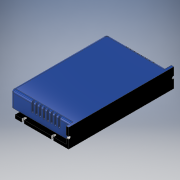
# Autodesk Inventor part: CopleyAccelus
Saved by Autodesk Inventor 2019 (Build 230136000, 136)
## iProperties
Created: 2019-05-13
Part Number: CopleyAccelus
Material: ABS Plastic
Document SubType Name: Modeling
Designer: Jorian Bruslind
Density: 1.06 g/cm^3
Appearance: Smooth - White
Author: Jorian Bruslind
Autodesk Inventor part; units mm, degrees
ref_plane "YZ Plane" through (0, 0, 0) normal (1, 0, 0) x (0, 1, 0)
ref_plane "XZ Plane" through (0, 0, 0) normal (0, 1, 0) x (-1, 0, 0)
sketch "Sketch1" plane through (0, 0, 0) normal (0, 1, 0) x (-1, 0, 0)
  line L0 (0, 0) -> (95, 0)
  line L1 (95, 0) -> (95, -152)
  line L2 (95, -152) -> (0, -152)
  line L3 (0, -152) -> (0, 0)
  dimension "d0" = 95
  dimension "d1" = 152
  constraints: 8 end point, 2 parallel, 1 horizontal, 1 perpendicular
  measures "d0" distance of L1.end L2.end
  measures "d1" distance of L0.end L1.end
extrude "Extrusion1" add sketch "Sketch1" along normal blind 25
sketch "Sketch2" plane through (0, 0, 0) normal (1, 0, 0) x (0, 0, -1)
  line L0 (0, 0) -> (0, -5)
  line L1 (0, -5) -> (-7.5, -5)
  line L2 (-7.5, -5) -> (159.5, -5)
  line L3 (159.5, -5) -> (159.5, 25)
  line L4 (159.5, 25) -> (-7.5, 25)
  line L5 (-7.5, 25) -> (-7.5, -5)
  point P0 (0, 25)
  dimension "d6" = 5
  dimension "d7" = 7.5
  dimension "d8" = 167
  dimension "d9" = 30
  constraints: 12 end point, 2 horizontal, 2 parallel, 1 perpendicular, 1 vertical
  measures "d6" distance of L0.start L0.end
  measures "d7" distance of L0.end L1.end
  measures "d8" distance of L4.end L3.end
  measures "d9" distance of L3.end L2.end
extrude "Extrusion2" add sketch "Sketch2" along normal blind 4
sketch "Sketch3" plane through (0, 0, 0) normal (-1, 0, 0) x (0, 0, 1)
  line L0 (7.5, 25) -> (7.5, -5) projected
  line L1 (-159.5, -5) -> (-159.5, 25) projected
  line L2 (7.5, -5) -> (-159.5, -5)
  line L3 (-159.5, -5) -> (-159.5, 0)
  line L4 (-159.5, 0) -> (7.5, 0)
  line L5 (7.5, 0) -> (7.5, -5)
  point P0 (0, 0)
  dimension "d12" = 5
  constraints: 8 end point, 2 parallel, 1 horizontal, 1 perpendicular, 1 point on line
  measures "d12" distance between parallel lines of L4 L2
extrude "Extrusion3" add sketch "Sketch3" along normal blind 81
sketch "Sketch4" plane through (4, -5, -159.5) normal (0, -1, 0) x (1, 0, 0)
  line L0 (-85, 0) -> (0, 0) projected
  line L1 (-85, 0) -> (-74.4, 0)
  line L2 (-74.4, 0) -> (-74.4, 3.5)
  arc A0 (-70.4, 3.5) -> (-74.4, 3.5) centre (-72.4, 3.5) ccw
  line L3 (-70.4, 3.5) -> (-70.4, 0)
  line L4 (-74.4, 0) -> (-70.4, 0)
  line L5 (-85, 0) -> (-85, 4)
  line L6 (-85, 0) -> (-85, 167) projected
  line L7 (-27.7, 0) -> (-27.7, 3.5)
  arc A1 (-23.7, 3.5) -> (-27.7, 3.5) centre (-25.7, 3.5) ccw
  line L8 (-23.7, 3.5) -> (-23.7, 0)
  line L9 (-27.7, 0) -> (-23.7, 0)
  line L10 (0, 0) -> (0, 167) projected
  line L11 (0, 0) -> (0, 83.5)
  line L12 (0, 83.5) -> (-10, 83.5)
  line L13 (-74.4, 167) -> (-74.4, 163.5)
  arc A2 (-74.4, 163.5) -> (-70.4, 163.5) centre (-72.4, 163.5) ccw
  line L14 (-70.4, 163.5) -> (-70.4, 167)
  line L15 (-74.4, 167) -> (-70.4, 167)
  line L16 (-27.7, 167) -> (-27.7, 163.5)
  arc A3 (-27.7, 163.5) -> (-23.7, 163.5) centre (-25.7, 163.5) ccw
  line L17 (-23.7, 163.5) -> (-23.7, 167)
  line L18 (-27.7, 167) -> (-23.7, 167)
  point P0 (-4, 159.5)
  dimension "d15" = 10.6
  dimension "d16" = 3.5
  dimension "d17" = 2
  dimension "d18" = 2
  dimension "d19" = 3.5
  dimension "d20" = 4
  dimension "d23" = 46.7
  dimension "d28" = 10
  constraints: 32 end point, 10 symmetric about line, 8 point on circle, 4 centre point, 3 point on line, 2 horizontal, 2 perpendicular, 1 midpoint, 1 vertical, 11 other
  measures "d15" distance of L0.start L1.end
  measures "d16" distance of L1.end L2.end
  measures "d17" radius of A0
  measures "d18" distance from line of L2 A0.centre
  measures "d19" distance of L3.start L3.end
  measures "d20" distance of L0.start L5.end
  measures "d23" distance of L1.end L7.start
  measures "d28" distance of L11.end L12.end
extrude "Extrusion4" cut sketch "Sketch4" against normal blind 5
fillet "Fillet1" radius 4 5 edges at (-47.5, 25, 0) (-47.5, 25, -152) (-95, 25, -76) (-95, 12.5, 0) (-95, 12.5, -152)
sketch "Sketch6" plane through (0, 25, 0) normal (0, 1, 0) x (1, 0, 0)
  line L0 (0, 0) -> (-18.5, 0)
  line L1 (-91, 0) -> (0, 0) projected
  line L2 (-18.5, 0) -> (-18.5, 1.5)
  arc A0 (-17, 1.5) -> (-20, 1.5) centre (-18.5, 1.5) ccw
  line L3 (-20, 1.5) -> (-20, 0)
  line L4 (-17, 1.5) -> (-17, 0)
  line L5 (-20, 0) -> (-17, 0)
  dimension "d41" = 18.5
  dimension "d42" = 1.5
  dimension "d43" = 1.5
  dimension "d44" = 1.5
  dimension "d45" = 1.5
  constraints: 10 end point, 3 perpendicular, 3 point on line, 2 point on circle, 1 centre point, 1 coincident, 1 collinear
  measures "d41" distance of L0.start L0.end
  measures "d42" distance of L0.end L2.end
  measures "d43" radius of A0
  measures "d44" distance of L3.start L3.end
  measures "d45" distance of L4.start L4.end
extrude "Extrusion6" cut sketch "Sketch6" against normal blind 14.5
sketch "Sketch7" plane through (-81, 0, 0) normal (0, 0, 1) x (1, 0, 0)
  line L0 (61, 10.5) -> (64, 10.5) projected
  arc A0 (61, 10.5) -> (64, 10.5) centre (62.5, 10.5) ccw
  line L1 (62.5, 10.5) -> (61, 10.5)
  line L2 (62.5, 10.5) -> (64, 10.5)
  point P0 (81, 0)
  constraints: 4 end point, 2 collinear, 2 point on circle, 1 centre point, 1 midpoint
extrude "Extrusion7" cut sketch "Sketch7" against normal blind 4.5
pattern_linear "Rectangular Pattern3" count 8 spacing 6 along (-1, 0, 0) of "Extrusion7", "Extrusion6"
ref_plane "Work Plane1" through (-81, 0, -76) normal (0, 0, 1) x (1, 0, 0)
mirror "Mirror1" about plane through (-81, 0, -76) normal (0, 0, 1) of "Extrusion7", "Extrusion6", "Rectangular Pattern3"
sketch "Sketch9" plane through (-95, 0, -148) normal (-1, 0, 0) x (0, 0, 1)
  line L0 (152, -5) -> (155.5, -5) projected
  line L1 (155.5, -5) -> (125, -5)
  line L2 (125, -5) -> (125, 5)
  line L3 (125, 5) -> (73.15, 5)
  line L4 (73.15, 5) -> (73.15, 18)
  line L5 (73.15, 18) -> (125, 18)
  line L6 (125, 18) -> (125, 5)
  line L7 (73.15, 5) -> (70.15, 5)
  line L8 (70.15, 5) -> (30.15, 5)
  line L9 (30.15, 5) -> (30.15, 18)
  line L10 (30.15, 18) -> (70.15, 18)
  line L11 (70.15, 18) -> (70.15, 5)
  point P0 (148, 0)
  dimension "d62" = 30.5
  dimension "d63" = 10
  dimension "d64" = 51.85
  dimension "d65" = 13
  dimension "d66" = 3
  dimension "d67" = 40
  dimension "d68" = 13
  constraints: 22 end point, 4 horizontal, 4 parallel, 3 perpendicular
  measures "d62" distance of L0.end L1.end
  measures "d63" distance of L1.end L2.end
  measures "d64" distance of L4.end L5.end
  measures "d65" distance of L3.end L4.end
  measures "d66" distance of L3.end L7.end
  measures "d67" distance of L9.end L10.end
  measures "d68" distance of L8.end L9.end
extrude "Extrusion8" cut sketch "Sketch9" against normal blind 6.3
sketch "Sketch10" plane through (0, 0, 0) normal (-1, 0, 0) x (0, 0, 1)
  line L0 (7.5, 25) -> (7.5, 0) projected
  line L1 (7.5, 25) -> (7.5, 12.5)
  line L2 (7.5, 12.5) -> (6.5, 12.5)
  line L3 (6.5, 12.5) -> (6.5, 10.5)
  arc A0 (6.5, 12.5) -> (6.5, 8.5) centre (6.5, 10.5) ccw
  line L4 (6.5, 10.5) -> (6.5, 8.5) construction
  line L5 (6.5, 10.5) -> (6.5, 12.5) construction
  line L6 (6.5, 8.5) -> (7.5, 8.5)
  line L7 (7.5, 12.5) -> (7.5, 8.5)
  line L8 (7.5, 25) -> (-76, 25)
  line L9 (-159.5, 25) -> (7.5, 25) projected
  line L10 (-76, 25) -> (-76, 17)
  line L11 (-148, 21) -> (-4, 21) projected
  line L12 (-76, 25) -> (-68, 25) construction
  line L13 (-159.5, 12.5) -> (-158.5, 12.5)
  arc A1 (-158.5, 8.5) -> (-158.5, 12.5) centre (-158.5, 10.5) ccw
  line L14 (-158.5, 8.5) -> (-159.5, 8.5)
  line L15 (-159.5, 12.5) -> (-159.5, 8.5)
  point P0 (0, 0)
  dimension "d71" = 1
  dimension "d72" = 2
  dimension "d73" = 180
  dimension "d74" = 8
  dimension "d75" = 90
  constraints: 26 end point, 5 symmetric about line, 4 perpendicular, 4 point on circle, 2 centre point, 2 horizontal, 2 midpoint, 1 coincident, 1 point on line, 1 vertical, 1 other
  measures "d71" distance of L1.end L2.end
  measures "d72" distance of L2.end L3.end
  measures "d73" angle of L5 L4
  measures "d74" distance of L8.end L10.end
  measures "d75" angle of L10 L12
extrude "Extrusion9" cut sketch "Sketch10" against normal blind 4
body "Solid1"
